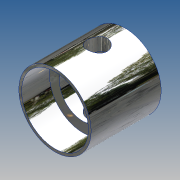
# Autodesk Inventor part: Kolben_ra8846s
Saved by Autodesk Inventor 2021 (Build 250183000, 183)
## iProperties
Created: 2020-11-17
Part Number: Kolben_ra8846s
Material: Aluminium 6061
Document SubType Name: Modeling
Designer: Ricardo a
Density: 2.7 g/cm^3
Appearance: Aluminium - flach
Description: Motor_Teil9_Kolben
Mass: 1.99187 g
Surface Area: 11.3377 cm^2
Volume: 0.737728 cm^3
Author: Sander
Revision Number: Rev00
Autodesk Inventor part; units mm, degrees
ref_plane "YZ-Ebene" through (0, 0, 0) normal (1, 0, 0) x (0, 1, 0)
ref_plane "XZ-Ebene" through (0, 0, 0) normal (0, 1, 0) x (-1, 0, 0)
ref_plane "XY-Ebene" through (0, 0, 0) normal (0, 0, 1) x (1, 0, 0)
sketch "Skizze1" plane through (0, 0, 0) normal (0, 0, 1) x (1, 0, 0)
  line L0 (-1.3, 0) -> (7.8, 0) projected
  line L1 (0, -2.52) -> (0, 15.12) projected
  line L2 (0, 12.6) -> (6.5, 12.6)
  line L3 (6.5, 12.6) -> (6.5, 0)
  line L4 (6, 0) -> (6, 5)
  line L5 (6, 5) -> (4.2, 5)
  line L6 (4.2, 5) -> (4.2, 10.8)
  line L7 (4.2, 10.8) -> (0, 10.8)
  point P0 (0, 0)
  dimension "d0" = 6.5
  dimension "d1" = 5
  dimension "d2" = 12.6
  dimension "d3" = 1.8
  dimension "d4" = 5.8
  dimension "d5" = 4.2
  dimension "d6" = 0.5
  constraints: 12 end point, 4 perpendicular, 3 point on line, 1 horizontal, 1 vertical
  measures "d0" distance of L2.start L2.end
  measures "d1" distance of L4.start L4.end
  measures "d2" distance of L2.end L3.end
  measures "d3" distance of L4.end L5.end
  measures "d4" distance of L5.end L6.end
  measures "d5" distance of L6.end L7.end
  measures "d6" distance between parallel lines of L3 L4
revolve "Umdrehung1" add sketch "Skizze1" angle 360 about axis through (0, -10, 0) along (0, 1, 0) contours L4 L5 L6 L7 L1 L2 L3 L0
sketch "Skizze2" plane through (0, 0, 0) normal (0, 0, 1) x (1, 0, 0)
  line L0 (6.5, 12.6) -> (-6.5, 12.6) projected
  line L1 (4.2, 10.8) -> (-4.2, 10.8) projected
  circle A0 centre (0, 7.6) radius 1.8
  point P0 (0, 0)
  dimension "d13" = 3.6
  dimension "d14" = 5
  constraints: 1 centre point, 1 vertical alignment
  measures "d13" diameter of A0
  measures "d14" distance from line of L0 A0.centre
extrude "Extrusion1" cut sketch "Skizze2" along normal through all both and the other way through all
